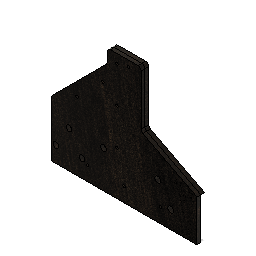
MountingPlate_v38 (Autodesk Fusion 360 design; units mm, degrees)
Autodesk Fusion 360 part; units mm, degrees
sketch "Sketch1" plane through (0, 0, 0) normal (0, 0, 1) x (1, 0, 0)
  line L0 (0, 0) -> (228, 0)
  line L1 (228, 0) -> (228, 110)
  line L2 (228, 110) -> (0, 110)
  line L3 (0, 110) -> (0, 0)
  line L4 (87.5, 27) -> (140.5, 27)
  line L5 (140.5, 27) -> (140.5, 197)
  line L6 (140.5, 197) -> (87.5, 197)
  line L7 (87.5, 197) -> (87.5, 27)
  line L8 (0, 88) -> (120.2082, 208.2082)
  line L9 (120.2082, 208.2082) -> (157.6848, 170.7315)
  line L10 (157.6848, 170.7315) -> (37.4767, 50.5233)
  line L11 (37.4767, 50.5233) -> (0, 88)
  line L12 (102.5, 197) -> (102.5, 27) construction
  line L13 (10.6066, 77.3934) -> (130.8148, 197.6016) construction
  circle A0 centre (102.5, 126) radius 1.95
  circle A1 centre (80.6102, 147.397) radius 1.95
  circle A2 centre (40.3051, 107.0919) radius 1.95
  circle A3 centre (102.5, 69) radius 1.95
  circle A4 centre (102.5, 183) radius 1.95
  circle A5 centre (120.9153, 187.7021) radius 1.95
  line L14 (0, 22.5) -> (228, 22.5) construction
  circle A6 centre (57, 22.5) radius 1.95
  circle A7 centre (114, 22.5) radius 1.95
  circle A8 centre (171, 22.5) radius 1.95
  line L15 (140.5, 110) -> (228, 65)
  line L16 (228, 65) -> (0, 65)
  line L17 (0, 57.985) -> (228, 57.985) construction
  circle A9 centre (81.53, 57.985) radius 4.5
  circle A10 centre (166.53, 57.985) radius 4.5
  circle A11 centre (187, 27.5) radius 4.5
  circle A12 centre (7.015, 25) radius 4.5
  line L18 (4.9497, 83.0503) -> (125.1579, 203.2584) construction
  circle A13 centre (54.8008, 132.9013) radius 3.5
  circle A14 centre (82.3779, 105.3241) radius 3.5
  line L19 (49.851, 137.851) -> (87.3277, 100.3744) construction
  circle A15 centre (133.5, 97.5) radius 3.5
  circle A16 centre (94.5, 97.5) radius 3.5
  circle A17 centre (48, 27.5) radius 4.5
  circle A18 centre (27.53, 57.985) radius 4.5
  point P0 (114, 27)
  point P1 (114, 110)
  dimension "d12" = 53
  dimension "d13" = 53
  dimension "d16" = 170
  dimension "d17" = 170
  dimension "d18" = 45
  dimension "d22" = 42
  dimension "d24" = 42
  dimension "d25" = 57
  dimension "d26" = 57
  dimension "d27" = 57
  dimension "d29" = 57
  dimension "d30" = 3.9
  dimension "d31" = 3.9
  dimension "d32" = 3.9
  dimension "d33" = 3.9
  dimension "d34" = 3.9
  dimension "d35" = 3.9
  dimension "d36" = 15
  dimension "d37" = 15
  dimension "d40" = 22.5
  dimension "d43" = 57
  dimension "d44" = 57
  dimension "d48" = 88
  dimension "d49" = 110
  dimension "d50" = 57
  dimension "d51" = 3.9
  dimension "d52" = 3.9
  dimension "d53" = 3.9
  dimension "d55" = 27
  dimension "d57" = 65
  dimension "d62" = 7.015
  dimension "d63" = 81.53
  dimension "d64" = 85
  dimension "d65" = 9
  dimension "d66" = 9
  dimension "d68" = 37.5
  dimension "d69" = 9
  dimension "d70" = 187
  dimension "d71" = 7.015
  dimension "d72" = 9
  dimension "d73" = 25
  dimension "d78" = 7
  dimension "d79" = 7
  dimension "d82" = 70.5
  dimension "d85" = 7
  dimension "d87" = 7
  dimension "d88" = 7
  dimension "d89" = 7
  dimension "d90" = 7
  dimension "d91" = 7
  dimension "d92" = 70.5
  dimension "d98" = 9
  dimension "d100" = 9
  dimension "d101" = 29.47
  dimension "d102" = 57.985
  dimension "d103" = 9
  constraint horizontal L0
  constraint vertical L1
  constraint horizontal L2
  constraint vertical L3
  constraint horizontal L4
  constraint vertical L5
  constraint horizontal L6
  constraint vertical L7
  constraint perpendicular L8 L9
  constraint parallel L8 L10
  constraint parallel L9 L11
  constraint coincident L12 A0.centre
  constraint coincident L13 A1.centre
  constraint coincident L13 A2.centre
  constraint coincident L12 A3.centre
  constraint coincident L12 A4.centre
  constraint coincident L13 A5.centre
  constraint coincident L6 L12.start
  constraint perpendicular L6 L12
  constraint coincident L4 L12.end
  constraint coincident L11 L13.start
  constraint coincident L9 L13.end
  constraint perpendicular L9 L13
  constraint coincident L0.start L3.end
  constraint coincident L3 L14.start
  constraint coincident L1 L14.end
  constraint perpendicular L1 L14
  constraint coincident L14 A6.centre
  constraint coincident L14 A8.centre
  constraint coincident L14 A7.centre
  constraint midpoint L14 A7.centre
  constraint coincident L4.start L7.end
  constraint midpoint L4 P0
  constraint midpoint L2 P1
  constraint vertical P0 P1
  constraint coincident L5 L15.start
  constraint coincident L2 L15.start
  constraint coincident L1 L15.end
  constraint coincident L3 L8.start
  constraint coincident L3 L16.end
  constraint perpendicular L3 L16
  constraint coincident L3 L17.start
  constraint coincident L1 L17.end
  constraint perpendicular L1 L17
  constraint coincident L17 A9.centre
  constraint coincident L17 A10.centre
  constraint coincident L11 L18.start
  constraint coincident L9 L18.end
  constraint perpendicular L9 L18
  constraint coincident L18 A13.centre
  constraint coincident L8 L19.start
  constraint perpendicular L18 L19
  constraint coincident L10 L19.end
  constraint coincident A13.centre L19
  constraint coincident A14.centre L19
  constraint horizontal A15.centre A16.centre
  constraint horizontal A11.centre A17.centre
  measures "d12" distance of L8.end L9.end
  measures "d13" distance of L5.end L6.end
  measures "d16" distance of L9.end L10.end
  measures "d17" distance of L4.end L5.end
  measures "d18" angle of L0 L10
  measures "d22" distance of L13.start A2.centre
  measures "d24" distance of L12.end A3.centre
  measures "d25" distance of A0.centre A3.centre
  measures "d26" distance of A1.centre A2.centre
  measures "d27" distance of A0.centre A4.centre
  measures "d29" distance of A1.centre A5.centre
  measures "d30" diameter of A3
  measures "d31" diameter of A0
  measures "d32" diameter of A4
  measures "d33" diameter of A2
  measures "d34" diameter of A1
  measures "d35" diameter of A5
  measures "d36" distance of L7 L12
  measures "d37" distance of L8 L13.end
  measures "d40" distance of L0 L14
  measures "d43" distance of A6.centre A7.centre
  measures "d44" distance of A7.centre A8.centre
  measures "d48" distance of L0 L8.start
  measures "d49" distance of L0 L2
  measures "d50" distance of L3 A6.centre
  measures "d51" diameter of A6
  measures "d52" diameter of A7
  measures "d53" diameter of A8
  measures "d55" distance of L0 P0
  measures "d57" distance of L0 L15.end
  measures "d62" distance of L16 L17
  measures "d63" distance of L3 A9.centre
  measures "d64" distance of A9.centre A10.centre
  measures "d65" diameter of A10
  measures "d66" diameter of A9
  measures "d68" distance of L16 A11.centre
  measures "d69" diameter of A11
  measures "d70" distance of L3 A11.centre
  measures "d71" distance of L3 A12.centre
  measures "d72" diameter of A12
  measures "d73" distance of L0 A12.centre
  measures "d78" distance of L8 L18
  measures "d79" diameter of A13
  measures "d82" distance of L11 A13.centre
  measures "d85" diameter of A14
  measures "d87" distance of L10 A14.centre
  measures "d88" diameter of A15
  measures "d89" diameter of A16
  measures "d90" distance of L5 A15.centre
  measures "d91" distance of L7 A16.centre
  measures "d92" distance of L4 A15.centre
  measures "d98" horizontal distance of A6.centre A17.centre
  measures "d100" diameter of A17
  measures "d101" horizontal distance of A6.centre A18.centre
  measures "d102" distance of L0 A18.centre
  measures "d103" diameter of A18
extrude "Extrude1" add sketch "Sketch1" along normal blind 6 contours L0 L1 L3 L4 L5 L7 L10 L11 L16 A18 | L3 L11 L16 | L5 L15 L16 | L2 L7 L8 L10 L11 L16 | L10 L11 L16 A18 | L2 L5 L7 L10 L16 | L2 L5 L10 | L4 L5 L7 L16 | L2 L7 L8 | L7 L10 L16 | L2 L7 L10 | L2 L5 L6 L7 L8 L9 L10 | L6 L7 L8 | L5 L6 L9 | A13 | A14 | A15 | A16 makes body 1
extrude "Extrude1'" add sketch "Sketch1" against normal blind 6 separate body contours L3 L11 L16 | L5 L15 L16 | L2 L7 L8 L10 L11 L16 | L2 L5 L7 L10 L16 | L2 L5 L10 | L2 L7 L8 | L7 L10 L16 | L2 L7 L10 | L2 L5 L6 L7 L8 L9 L10 | L6 L7 L8 | L5 L6 L9 makes body 2 in component "Component"
fillet "Fillet1" radius 5 5 edges at (0, 88, 3) (87.5, 197, 3) (140.5, 197, 3) (140.5, 110, 3) (87.5, 175.5, 3) on bodies 1
fillet "Fillet1'" radius 5 5 edges at (0, 88, -3) (87.5, 197, -3) (140.5, 197, -3) (140.5, 110, -3) (87.5, 175.5, -3) on bodies 2 in component "Component"
component "Component" placed x (1, 0, 0) y (0, 1, 0) z (0, 0, 1) at (0, 0, 0)
equation "d13 = d12"
equation "d17 = d16"
equation "d24 = d22"
equation "d26 = d25"
equation "d27 = d25"
equation "d29 = d26"
equation "d31 = d30"
equation "d32 = d30"
equation "d33 = d30"
equation "d34 = d30"
equation "d35 = d30"
equation "d37 = d36"
equation "d44 = d43"
equation "d48 = 96 mm - 8 mm"
equation "d50 = d43"
equation "d52 = d51"
equation "d53 = d51"
equation "d66 = d65"
equation "d69 = d66"
equation "d70 = 203 mm - 16 mm"
equation "d72 = d66"
equation "d85 = d79"
equation "d87 = d78"
equation "d89 = d88"
equation "d91 = d90"
equation "d92 = d82"
equation "d100 = d72"
equation "d103 = d72"
